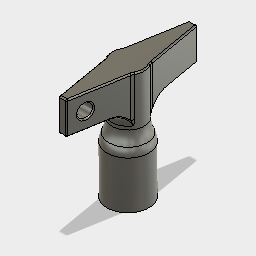
tuningKey (Autodesk Fusion 360 design; units mm, degrees)
Autodesk Fusion 360 part; units mm, degrees
sketch "スケッチ1" plane through (0, 0, 0) normal (0, 1, 0) x (1, 0, 0)
  line L0 (5.25, 3.0311) -> (0, 6.0622)
  line L1 (0, 6.0622) -> (-5.25, 3.0311)
  line L2 (-5.25, 3.0311) -> (-5.25, -3.0311)
  line L3 (-5.25, -3.0311) -> (0, -6.0622)
  line L4 (0, -6.0622) -> (5.25, -3.0311)
  line L5 (5.25, -3.0311) -> (5.25, 3.0311)
  circle A0 centre (0, 0) radius 8
  dimension "d1" = 16
  measures "d1" diameter of A0
extrude "押し出し1" add sketch "スケッチ1" along normal blind 30 makes body 1
sketch "スケッチ2" plane through (0, 30, 0) normal (0, 1, 0) x (-1, 0, 0)
  line L0 (-5.25, -3.0311) -> (-5.25, 3.0311)
  line L1 (-5.25, 3.0311) -> (0, 6.0622)
  line L2 (0, 6.0622) -> (5.25, 3.0311)
  line L3 (5.25, 3.0311) -> (5.25, -3.0311)
  line L4 (5.25, -3.0311) -> (0, -6.0622)
  line L5 (0, -6.0622) -> (-5.25, -3.0311)
  circle A0 centre (0, 0) radius 8
extrude "押し出し2" add sketch "スケッチ2" against normal blind 15 contours L0 L1 L2 L3 L4 L5 bodies 1
sketch "スケッチ3" plane through (0, 30, 0) normal (0, 1, 0) x (-1, 0, 0)
  circle A0 centre (0, 0) radius 8
  circle A1 centre (0, 0) radius 6.25
  dimension "d6" = 12.5
  measures "d6" diameter of A1
extrude "押し出し3" cut sketch "スケッチ3" against normal blind 10 bodies 1
sketch "スケッチ4" plane through (0, 0, 0) normal (1, 0, 0) x (0, 0, -1)
  line L0 (0, 30) -> (0, 45)
  line L1 (0, 45) -> (25, 45)
  line L2 (0, 45) -> (-25, 45)
  line L3 (-25, 45) -> (-25, 32.5)
  line L4 (-25, 32.5) -> (25, 32.5)
  line L5 (25, 32.5) -> (25, 45)
  point P0 (0, 30)
  dimension "d14" = 12.5
  measures "d14" distance of L2.end L3.end
extrude "押し出し4" add sketch "スケッチ4" along normal mid plane 11 separate body makes body 2
chamfer "面取り1" distance 23 distance2 4 4 edges at (5.5, 38.75, 25) (-5.5, 38.75, 25) (-5.5, 38.75, -25) (5.5, 38.75, -25) measured on face at (5.5, 36.6667, -8.3333) measured on face at (-5.5, 36.6667, -8.3333) measured on face at (-5.5, 36.6667, -8.3333) measured on face at (5.5, 36.6667, -8.3333) on bodies 2
move_face "面をオフセット1" offset 15 1 faces at (3.0203, 30, 1.0762) on bodies 1
combine "結合1" operation add target body 2 tool bodies 1
fillet "フィレット3" radius 12 1 edges at (5.827, 20, -2.2601) on bodies 2
fillet "フィレット4" radius 7.5 1 edges at (-7.4586, 20, -2.8929) on bodies 2
fillet "フィレット5" radius 5 3 edges at (0, 32.5, -6.25) (0, 32.5, 6.25) (0, 32.5, 6.25) on bodies 2
sketch "スケッチ5" plane through (0, 0, 0) normal (0, 1, 0) x (1, 0, 0)
sketch "スケッチ6" plane through (0, 0, 0) normal (1, 0, 0) x (0, 0, -1)
  line L0 (-3.15, 45) -> (3.15, 45)
  line L1 (0, 0) -> (0, 45)
  line L2 (-24, 32.5) -> (-10.8426, 32.5)
  line L3 (-14.985, 32.5) -> (0, 32.5)
  line L4 (0, 32.5) -> (0, 38.75)
  circle A0 centre (0, 38.75) radius 2.5
  line L5 (-25, 44) -> (-25, 33.5)
  line L6 (0, 38.75) -> (-25, 38.75)
  line L7 (-25, 38.75) -> (-18.75, 38.75)
  circle A1 centre (-18.75, 38.75) radius 2.5
  dimension "d30" = 6.25
  dimension "d31" = 5
  dimension "d32" = 6.25
  dimension "d33" = 5
  measures "d30" distance of L3.end L4.end
  measures "d31" diameter of A0
  measures "d32" distance of L6.end L7.end
  measures "d33" diameter of A1
extrude "押し出し5" cut sketch "スケッチ6" along normal mid plane 34 contours L6 L7 A1 | L6 L7 A1 bodies 2
fillet "フィレット16" radius 0.5 8 edges at (-2.7603, 32.5, -17.7535) (-4.7835, 31.0877, -6.1201) (4.7835, 31.0877, -6.1201) (2.7603, 32.5, -17.7535) (2.7603, 32.5, 17.7535) (4.7835, 31.0877, 6.1201) (-2.7603, 32.5, 17.7535) (-4.7835, 31.0877, 6.1201) on bodies 2
fillet "フィレット17" radius 4 8 edges at (5.2468, 27.8361, 3.3962) (5.261, 36.5906, 3.374) (5.261, 36.5906, -3.374) (5.2468, 27.8361, -3.3961) (-5.261, 36.5906, 3.374) (-5.2468, 27.8361, 3.3961) (-5.2468, 27.8361, -3.3962) (-5.261, 36.5906, -3.374) on bodies 2
fillet "フィレット18" radius 0.5 10 edges at (-3.3202, 45, 14.534) (-5.2934, 45, 3.4678) (-6.25, 45, 0) (-5.2934, 45, -3.4678) (-3.3202, 45, -14.534) (3.3202, 45, -14.534) (5.2934, 45, -3.4678) (6.25, 45, 0) (5.2934, 45, 3.4678) (3.3202, 45, 14.534) on bodies 2
fillet "フィレット19" radius 0.5 16 edges at (0, 45, -25) (-1.3514, 44.8536, -25) (-1.5, 38.75, -25) (-1.3514, 32.6464, -25) (0, 32.5, -25) (1.3514, 32.6464, -25) (1.5, 38.75, -25) (1.3514, 44.8536, -25) (-1.3514, 32.6464, 25) (0, 32.5, 25) (1.3514, 32.6464, 25) (1.5, 38.75, 25) (1.3514, 44.8536, 25) (0, 45, 25) (-1.3514, 44.8536, 25) (-1.5, 38.75, 25) on bodies 2
fillet "フィレット20" radius 0.5 2 edges at (-2.1522, 38.75, 21.25) (2.1522, 38.75, 21.25) on bodies 2
